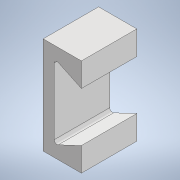
# Autodesk Inventor part: dovetail insert
Saved by Autodesk Inventor 2022 (Build 260153000, 153)
## iProperties
Created: 2022-11-13
Part Number: dovetail insert
Material: Generic
Document SubType Name: Modeling
Designer: efred
Density: 1 g/cm^3
Appearance: Default
Author: efred
Autodesk Inventor part; units mm, degrees
ref_plane "YZ Plane" through (0, 0, 0) normal (1, 0, 0) x (0, 1, 0)
ref_plane "XZ Plane" through (0, 0, 0) normal (0, 1, 0) x (-1, 0, 0)
ref_plane "XY Plane" through (0, 0, 0) normal (0, 0, 1) x (1, 0, 0)
sketch "Sketch1" plane through (0, 0, 0) normal (0, 0, 1) x (1, 0, 0)
  circle A0 centre (2.8524, -17.9) radius 2 projected
  circle A1 centre (18.8524, -17.9) radius 2 projected
  circle A2 centre (18.8524, 17.9) radius 2 projected
  circle A3 centre (2.8524, 17.9) radius 2 projected
  arc A4 (3.1135, 5.1575) -> (3.0054, 10.8589) centre (-1.0472, 7.9303) ccw projected
  arc A5 (3.1135, 5.1575) -> (2.4476, 3.9812) centre (10.8524, 0) ccw projected
  line L0 (2.4476, 3.9812) -> (-1.0195, 5.6235) projected
  line L1 (-2.4476, 4.7198) -> (-2.4476, -4.7198) projected
  line L2 (-1.0195, -5.6235) -> (2.4476, -3.9812) projected
  arc A6 (2.4476, -3.9812) -> (3.1135, -5.1575) centre (10.8524, 0) ccw projected
  arc A7 (3.0054, -10.8589) -> (3.1135, -5.1575) centre (-1.0472, -7.9303) ccw projected
  line L3 (-0.3897, -15.5572) -> (3.0054, -10.8589) projected
  arc A8 (-0.3897, -15.5572) -> (6.4079, -19.7325) centre (2.8524, -17.9) ccw projected
  arc A9 (15.2968, -19.7325) -> (6.4079, -19.7325) centre (10.8524, -22.0231) ccw projected
  arc A10 (15.2968, -19.7325) -> (22.0945, -15.5572) centre (18.8524, -17.9) ccw projected
  line L4 (22.0945, -15.5572) -> (18.6993, -10.8589) projected
  arc A11 (18.3102, -5.6345) -> (18.6993, -10.8589) centre (22.752, -7.9303) ccw projected
  line L5 (32.1524, -5.6345) -> (18.3102, -5.6345) projected
  line L6 (32.1524, 5.6345) -> (32.1524, -5.6345) projected
  line L7 (32.1524, 5.6345) -> (18.3102, 5.6345) projected
  arc A12 (18.6993, 10.8589) -> (18.3102, 5.6345) centre (22.752, 7.9303) ccw projected
  line L8 (18.6993, 10.8589) -> (22.0945, 15.5572) projected
  arc A13 (22.0945, 15.5572) -> (15.2968, 19.7325) centre (18.8524, 17.9) ccw projected
  arc A14 (6.4079, 19.7325) -> (15.2968, 19.7325) centre (10.8524, 22.0231) ccw projected
  arc A15 (6.4079, 19.7325) -> (-0.3897, 15.5572) centre (2.8524, 17.9) ccw projected
  line L9 (3.0054, 10.8589) -> (-0.3897, 15.5572) projected
  circle A16 centre (10.8524, 0) radius 1.5 projected
  line L10 (2.2476, 4.2972) -> (-2.6476, 6.616)
  line L11 (-2.6476, 6.616) -> (-2.6476, -6.616)
  line L12 (-2.6476, -6.616) -> (2.2476, -4.2972)
  line L13 (0, 0) -> (10.8524, 0) construction
  line L14 (2.2476, 4.2972) -> (2.2476, 8.616)
  line L15 (2.2476, 8.616) -> (-4.6476, 8.616)
  line L16 (-4.6476, 8.616) -> (-4.6476, -8.616)
  line L17 (-4.6476, -8.616) -> (2.2476, -8.616)
  line L18 (2.2476, -8.616) -> (2.2476, -4.2972)
  arc A17 (-2.4476, -4.7198) -> (-1.0195, -5.6235) centre (-1.4476, -4.7198) ccw projected
  arc A18 (-1.0195, 5.6235) -> (-2.4476, 4.7198) centre (-1.4476, 4.7198) ccw projected
  dimension "d0" = 0.2
  dimension "d1" = 0.2
  dimension "d2" = 0.2
  dimension "d3" = 2
  dimension "d4" = 2
  constraints: 18 end point, 4 perpendicular, 2 parallel, 2 vertical, 1 point on line, 1 symmetric about line, 3 other
  measures "d0" distance between parallel lines of L0 L10
  measures "d1" distance between parallel lines of L1 L11
  measures "d2" horizontal distance of L0.start L10.start
  measures "d3" distance between parallel lines of L11 L16
  measures "d4" distance from line of L10.end L15
extrude "Extrusion1" add sketch "Sketch1" against normal blind 10 contours L10 L11 L12 L18 L17 L16 L15 L14
fillet "Fillet1" radius 1 2 edges at (-2.6476, -6.616, -5) (-2.6476, 6.616, -5)
body "Solid1"
